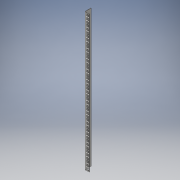
# Autodesk Inventor part: 15U_rack_strip
Saved by Autodesk Inventor 2016 (Build 200138000, 138)
## iProperties
Created: 2016-10-05
Part Number: 15U_rack_strip
Material: Generic
Document SubType Name: Sheet Metal
Designer: gmmar
Density: 1 g/cm^3
Sheet Metal Rule: Default
Appearance: Default
Author: gmmar
Autodesk Inventor part; units mm, degrees
ref_plane "YZ Plane" through (0, 0, 0) normal (1, 0, 0) x (0, 1, 0)
ref_plane "XZ Plane" through (0, 0, 0) normal (0, 1, 0) x (-1, 0, 0)
ref_plane "XY Plane" through (0, 0, 0) normal (0, 0, 1) x (1, 0, 0)
sketch "Sketch1" plane through (0, 0, 0) normal (0, 0, 1) x (1, 0, 0)
  line L0 (-22.7601, 80.4963) -> (27.2399, 80.4963)
  line L1 (27.2399, 80.4963) -> (27.2399, -590.5037)
  line L2 (27.2399, -590.5037) -> (-22.7601, -590.5037)
  line L3 (-22.7601, -590.5037) -> (-22.7601, 80.4963)
  line L4 (25.2399, 77.4963) -> (15.2399, 77.4963)
  line L5 (15.2399, 77.4963) -> (15.2399, 67.4963)
  line L6 (15.2399, 67.4963) -> (25.2399, 67.4963)
  line L7 (25.2399, 67.4963) -> (25.2399, 77.4963)
  line L8 (15.2399, 61.6213) -> (25.2399, 61.6213)
  line L9 (25.2399, 61.6213) -> (25.2399, 51.6213)
  line L10 (25.2399, 51.6213) -> (15.2399, 51.6213)
  line L11 (15.2399, 51.6213) -> (15.2399, 61.6213)
  line L12 (15.2399, 45.7463) -> (25.2399, 45.7463)
  line L13 (25.2399, 45.7463) -> (25.2399, 35.7463)
  line L14 (25.2399, 35.7463) -> (15.2399, 35.7463)
  line L15 (15.2399, 35.7463) -> (15.2399, 45.7463)
  line L16 (15.8399, 79.6042) -> (24.6399, 79.6042)
  line L17 (25.2399, 79.0042) -> (25.2399, 78.6883)
  line L18 (24.6399, 78.0883) -> (15.8399, 78.0883)
  line L19 (15.2399, 78.6883) -> (15.2399, 79.0042)
  line L20 (15.2399, 79.6042) -> (25.2399, 78.0883) construction
  line L21 (25.2399, 79.6042) -> (15.2399, 78.0883) construction
  arc A0 (15.8399, 79.6042) -> (15.2399, 79.0042) centre (15.8399, 79.0042) ccw
  arc A1 (15.2399, 78.6883) -> (15.8399, 78.0883) centre (15.8399, 78.6883) ccw
  arc A2 (24.6399, 78.0883) -> (25.2399, 78.6883) centre (24.6399, 78.6883) ccw
  arc A3 (25.2399, 79.0042) -> (24.6399, 79.6042) centre (24.6399, 79.0042) ccw
  circle A4 centre (-11.0789, 56.1463) radius 2.6
  line L22 (15.2399, 17.1713) -> (25.2399, 17.1713)
  circle A5 centre (-11.0789, 11.6963) radius 2.6
  line L23 (15.2399, 7.1713) -> (15.2399, 17.1713)
  line L24 (25.2399, 17.1713) -> (25.2399, 7.1713)
  line L25 (25.2399, 7.1713) -> (15.2399, 7.1713)
  line L26 (15.2399, 1.2963) -> (25.2399, 1.2963)
  line L27 (15.2399, -8.7037) -> (15.2399, 1.2963)
  line L28 (25.2399, -8.7037) -> (15.2399, -8.7037)
  line L29 (25.2399, 1.2963) -> (25.2399, -8.7037)
  line L30 (25.2399, 33.0463) -> (15.2399, 33.0463)
  line L31 (15.2399, 33.0463) -> (15.2399, 23.0463)
  line L32 (15.2399, 23.0463) -> (25.2399, 23.0463)
  line L33 (25.2399, 23.0463) -> (25.2399, 33.0463)
  line L34 (25.2399, 34.5542) -> (25.2399, 34.2383)
  arc A6 (25.2399, 34.5542) -> (24.6399, 35.1542) centre (24.6399, 34.5542) ccw
  arc A7 (24.6399, 33.6383) -> (25.2399, 34.2383) centre (24.6399, 34.2383) ccw
  line L35 (24.6399, 33.6383) -> (15.8399, 33.6383)
  arc A8 (15.2399, 34.2383) -> (15.8399, 33.6383) centre (15.8399, 34.2383) ccw
  line L36 (15.2399, 35.1542) -> (25.2399, 33.6383) construction
  line L37 (25.2399, 35.1542) -> (15.2399, 33.6383) construction
  line L38 (15.8399, 35.1542) -> (24.6399, 35.1542)
  line L39 (15.2399, 34.2383) -> (15.2399, 34.5542)
  arc A9 (15.8399, 35.1542) -> (15.2399, 34.5542) centre (15.8399, 34.5542) ccw
  line L40 (15.2399, -27.2787) -> (25.2399, -27.2787)
  circle A10 centre (-11.0789, -32.7537) radius 2.6
  line L41 (15.2399, -37.2787) -> (15.2399, -27.2787)
  line L42 (25.2399, -27.2787) -> (25.2399, -37.2787)
  line L43 (25.2399, -37.2787) -> (15.2399, -37.2787)
  line L44 (15.2399, -43.1537) -> (25.2399, -43.1537)
  line L45 (15.2399, -53.1537) -> (15.2399, -43.1537)
  line L46 (25.2399, -53.1537) -> (15.2399, -53.1537)
  line L47 (25.2399, -43.1537) -> (25.2399, -53.1537)
  line L48 (25.2399, -11.4037) -> (15.2399, -11.4037)
  line L49 (15.2399, -11.4037) -> (15.2399, -21.4037)
  line L50 (15.2399, -21.4037) -> (25.2399, -21.4037)
  line L51 (25.2399, -21.4037) -> (25.2399, -11.4037)
  line L52 (25.2399, -9.8958) -> (25.2399, -10.2117)
  arc A11 (25.2399, -9.8958) -> (24.6399, -9.2958) centre (24.6399, -9.8958) ccw
  arc A12 (24.6399, -10.8117) -> (25.2399, -10.2117) centre (24.6399, -10.2117) ccw
  line L53 (24.6399, -10.8117) -> (15.8399, -10.8117)
  arc A13 (15.2399, -10.2117) -> (15.8399, -10.8117) centre (15.8399, -10.2117) ccw
  line L54 (15.2399, -9.2958) -> (25.2399, -10.8117) construction
  line L55 (25.2399, -9.2958) -> (15.2399, -10.8117) construction
  line L56 (15.8399, -9.2958) -> (24.6399, -9.2958)
  line L57 (15.2399, -10.2117) -> (15.2399, -9.8958)
  arc A14 (15.8399, -9.2958) -> (15.2399, -9.8958) centre (15.8399, -9.8958) ccw
  line L58 (15.2399, -71.7287) -> (25.2399, -71.7287)
  circle A15 centre (-11.0789, -77.2037) radius 2.6
  line L59 (15.2399, -81.7287) -> (15.2399, -71.7287)
  line L60 (25.2399, -71.7287) -> (25.2399, -81.7287)
  line L61 (25.2399, -81.7287) -> (15.2399, -81.7287)
  line L62 (15.2399, -87.6037) -> (25.2399, -87.6037)
  line L63 (15.2399, -97.6037) -> (15.2399, -87.6037)
  line L64 (25.2399, -97.6037) -> (15.2399, -97.6037)
  line L65 (25.2399, -87.6037) -> (25.2399, -97.6037)
  line L66 (25.2399, -55.8537) -> (15.2399, -55.8537)
  line L67 (15.2399, -55.8537) -> (15.2399, -65.8537)
  line L68 (15.2399, -65.8537) -> (25.2399, -65.8537)
  line L69 (25.2399, -65.8537) -> (25.2399, -55.8537)
  line L70 (25.2399, -54.3458) -> (25.2399, -54.6617)
  arc A16 (25.2399, -54.3458) -> (24.6399, -53.7458) centre (24.6399, -54.3458) ccw
  arc A17 (24.6399, -55.2617) -> (25.2399, -54.6617) centre (24.6399, -54.6617) ccw
  line L71 (24.6399, -55.2617) -> (15.8399, -55.2617)
  arc A18 (15.2399, -54.6617) -> (15.8399, -55.2617) centre (15.8399, -54.6617) ccw
  line L72 (15.2399, -53.7458) -> (25.2399, -55.2617) construction
  line L73 (25.2399, -53.7458) -> (15.2399, -55.2617) construction
  line L74 (15.8399, -53.7458) -> (24.6399, -53.7458)
  line L75 (15.2399, -54.6617) -> (15.2399, -54.3458)
  arc A19 (15.8399, -53.7458) -> (15.2399, -54.3458) centre (15.8399, -54.3458) ccw
  line L76 (15.2399, -116.1787) -> (25.2399, -116.1787)
  circle A20 centre (-11.0789, -121.6537) radius 2.6
  line L77 (15.2399, -126.1787) -> (15.2399, -116.1787)
  line L78 (25.2399, -116.1787) -> (25.2399, -126.1787)
  line L79 (25.2399, -126.1787) -> (15.2399, -126.1787)
  line L80 (15.2399, -132.0537) -> (25.2399, -132.0537)
  line L81 (15.2399, -142.0537) -> (15.2399, -132.0537)
  line L82 (25.2399, -142.0537) -> (15.2399, -142.0537)
  line L83 (25.2399, -132.0537) -> (25.2399, -142.0537)
  line L84 (25.2399, -100.3037) -> (15.2399, -100.3037)
  line L85 (15.2399, -100.3037) -> (15.2399, -110.3037)
  line L86 (15.2399, -110.3037) -> (25.2399, -110.3037)
  line L87 (25.2399, -110.3037) -> (25.2399, -100.3037)
  line L88 (25.2399, -98.7958) -> (25.2399, -99.1117)
  arc A21 (25.2399, -98.7958) -> (24.6399, -98.1958) centre (24.6399, -98.7958) ccw
  arc A22 (24.6399, -99.7117) -> (25.2399, -99.1117) centre (24.6399, -99.1117) ccw
  line L89 (24.6399, -99.7117) -> (15.8399, -99.7117)
  arc A23 (15.2399, -99.1117) -> (15.8399, -99.7117) centre (15.8399, -99.1117) ccw
  line L90 (15.2399, -98.1958) -> (25.2399, -99.7117) construction
  line L91 (25.2399, -98.1958) -> (15.2399, -99.7117) construction
  line L92 (15.8399, -98.1958) -> (24.6399, -98.1958)
  line L93 (15.2399, -99.1117) -> (15.2399, -98.7958)
  arc A24 (15.8399, -98.1958) -> (15.2399, -98.7958) centre (15.8399, -98.7958) ccw
  line L94 (15.2399, -160.6287) -> (25.2399, -160.6287)
  circle A25 centre (-11.0789, -166.1037) radius 2.6
  line L95 (15.2399, -170.6287) -> (15.2399, -160.6287)
  line L96 (25.2399, -160.6287) -> (25.2399, -170.6287)
  line L97 (25.2399, -170.6287) -> (15.2399, -170.6287)
  line L98 (15.2399, -176.5037) -> (25.2399, -176.5037)
  line L99 (15.2399, -186.5037) -> (15.2399, -176.5037)
  line L100 (25.2399, -186.5037) -> (15.2399, -186.5037)
  line L101 (25.2399, -176.5037) -> (25.2399, -186.5037)
  line L102 (25.2399, -144.7537) -> (15.2399, -144.7537)
  line L103 (15.2399, -144.7537) -> (15.2399, -154.7537)
  line L104 (15.2399, -154.7537) -> (25.2399, -154.7537)
  line L105 (25.2399, -154.7537) -> (25.2399, -144.7537)
  line L106 (25.2399, -143.2458) -> (25.2399, -143.5617)
  arc A26 (25.2399, -143.2458) -> (24.6399, -142.6458) centre (24.6399, -143.2458) ccw
  arc A27 (24.6399, -144.1617) -> (25.2399, -143.5617) centre (24.6399, -143.5617) ccw
  line L107 (24.6399, -144.1617) -> (15.8399, -144.1617)
  arc A28 (15.2399, -143.5617) -> (15.8399, -144.1617) centre (15.8399, -143.5617) ccw
  line L108 (15.2399, -142.6458) -> (25.2399, -144.1617) construction
  line L109 (25.2399, -142.6458) -> (15.2399, -144.1617) construction
  line L110 (15.8399, -142.6458) -> (24.6399, -142.6458)
  line L111 (15.2399, -143.5617) -> (15.2399, -143.2458)
  arc A29 (15.8399, -142.6458) -> (15.2399, -143.2458) centre (15.8399, -143.2458) ccw
  line L112 (15.2399, -205.0787) -> (25.2399, -205.0787)
  circle A30 centre (-11.0789, -210.5537) radius 2.6
  line L113 (15.2399, -215.0787) -> (15.2399, -205.0787)
  line L114 (25.2399, -205.0787) -> (25.2399, -215.0787)
  line L115 (25.2399, -215.0787) -> (15.2399, -215.0787)
  line L116 (15.2399, -220.9537) -> (25.2399, -220.9537)
  line L117 (15.2399, -230.9537) -> (15.2399, -220.9537)
  line L118 (25.2399, -230.9537) -> (15.2399, -230.9537)
  line L119 (25.2399, -220.9537) -> (25.2399, -230.9537)
  line L120 (25.2399, -189.2037) -> (15.2399, -189.2037)
  line L121 (15.2399, -189.2037) -> (15.2399, -199.2037)
  line L122 (15.2399, -199.2037) -> (25.2399, -199.2037)
  line L123 (25.2399, -199.2037) -> (25.2399, -189.2037)
  line L124 (25.2399, -187.6958) -> (25.2399, -188.0117)
  arc A31 (25.2399, -187.6958) -> (24.6399, -187.0958) centre (24.6399, -187.6958) ccw
  arc A32 (24.6399, -188.6117) -> (25.2399, -188.0117) centre (24.6399, -188.0117) ccw
  line L125 (24.6399, -188.6117) -> (15.8399, -188.6117)
  arc A33 (15.2399, -188.0117) -> (15.8399, -188.6117) centre (15.8399, -188.0117) ccw
  line L126 (15.2399, -187.0958) -> (25.2399, -188.6117) construction
  line L127 (25.2399, -187.0958) -> (15.2399, -188.6117) construction
  line L128 (15.8399, -187.0958) -> (24.6399, -187.0958)
  line L129 (15.2399, -188.0117) -> (15.2399, -187.6958)
  arc A34 (15.8399, -187.0958) -> (15.2399, -187.6958) centre (15.8399, -187.6958) ccw
  line L130 (15.2399, -249.5287) -> (25.2399, -249.5287)
  circle A35 centre (-11.0789, -255.0037) radius 2.6
  line L131 (15.2399, -259.5287) -> (15.2399, -249.5287)
  line L132 (25.2399, -249.5287) -> (25.2399, -259.5287)
  line L133 (25.2399, -259.5287) -> (15.2399, -259.5287)
  line L134 (15.2399, -265.4037) -> (25.2399, -265.4037)
  line L135 (15.2399, -275.4037) -> (15.2399, -265.4037)
  line L136 (25.2399, -275.4037) -> (15.2399, -275.4037)
  line L137 (25.2399, -265.4037) -> (25.2399, -275.4037)
  line L138 (25.2399, -233.6537) -> (15.2399, -233.6537)
  line L139 (15.2399, -233.6537) -> (15.2399, -243.6537)
  line L140 (15.2399, -243.6537) -> (25.2399, -243.6537)
  line L141 (25.2399, -243.6537) -> (25.2399, -233.6537)
  line L142 (25.2399, -232.1458) -> (25.2399, -232.4617)
  arc A36 (25.2399, -232.1458) -> (24.6399, -231.5458) centre (24.6399, -232.1458) ccw
  arc A37 (24.6399, -233.0617) -> (25.2399, -232.4617) centre (24.6399, -232.4617) ccw
  line L143 (24.6399, -233.0617) -> (15.8399, -233.0617)
  arc A38 (15.2399, -232.4617) -> (15.8399, -233.0617) centre (15.8399, -232.4617) ccw
  line L144 (15.2399, -231.5458) -> (25.2399, -233.0617) construction
  line L145 (25.2399, -231.5458) -> (15.2399, -233.0617) construction
  line L146 (15.8399, -231.5458) -> (24.6399, -231.5458)
  line L147 (15.2399, -232.4617) -> (15.2399, -232.1458)
  arc A39 (15.8399, -231.5458) -> (15.2399, -232.1458) centre (15.8399, -232.1458) ccw
  line L148 (15.2399, -293.9787) -> (25.2399, -293.9787)
  circle A40 centre (-11.0789, -299.4537) radius 2.6
  line L149 (15.2399, -303.9787) -> (15.2399, -293.9787)
  line L150 (25.2399, -293.9787) -> (25.2399, -303.9787)
  line L151 (25.2399, -303.9787) -> (15.2399, -303.9787)
  line L152 (15.2399, -309.8537) -> (25.2399, -309.8537)
  line L153 (15.2399, -319.8537) -> (15.2399, -309.8537)
  line L154 (25.2399, -319.8537) -> (15.2399, -319.8537)
  line L155 (25.2399, -309.8537) -> (25.2399, -319.8537)
  line L156 (25.2399, -278.1037) -> (15.2399, -278.1037)
  line L157 (15.2399, -278.1037) -> (15.2399, -288.1037)
  line L158 (15.2399, -288.1037) -> (25.2399, -288.1037)
  line L159 (25.2399, -288.1037) -> (25.2399, -278.1037)
  line L160 (25.2399, -276.5958) -> (25.2399, -276.9117)
  arc A41 (25.2399, -276.5958) -> (24.6399, -275.9958) centre (24.6399, -276.5958) ccw
  arc A42 (24.6399, -277.5117) -> (25.2399, -276.9117) centre (24.6399, -276.9117) ccw
  line L161 (24.6399, -277.5117) -> (15.8399, -277.5117)
  arc A43 (15.2399, -276.9117) -> (15.8399, -277.5117) centre (15.8399, -276.9117) ccw
  line L162 (15.2399, -275.9958) -> (25.2399, -277.5117) construction
  line L163 (25.2399, -275.9958) -> (15.2399, -277.5117) construction
  line L164 (15.8399, -275.9958) -> (24.6399, -275.9958)
  line L165 (15.2399, -276.9117) -> (15.2399, -276.5958)
  arc A44 (15.8399, -275.9958) -> (15.2399, -276.5958) centre (15.8399, -276.5958) ccw
  line L166 (15.2399, -338.4287) -> (25.2399, -338.4287)
  circle A45 centre (-11.0789, -343.9037) radius 2.6
  line L167 (15.2399, -348.4287) -> (15.2399, -338.4287)
  line L168 (25.2399, -338.4287) -> (25.2399, -348.4287)
  line L169 (25.2399, -348.4287) -> (15.2399, -348.4287)
  line L170 (15.2399, -354.3037) -> (25.2399, -354.3037)
  line L171 (15.2399, -364.3037) -> (15.2399, -354.3037)
  line L172 (25.2399, -364.3037) -> (15.2399, -364.3037)
  line L173 (25.2399, -354.3037) -> (25.2399, -364.3037)
  line L174 (25.2399, -322.5537) -> (15.2399, -322.5537)
  line L175 (15.2399, -322.5537) -> (15.2399, -332.5537)
  line L176 (15.2399, -332.5537) -> (25.2399, -332.5537)
  line L177 (25.2399, -332.5537) -> (25.2399, -322.5537)
  line L178 (25.2399, -321.0458) -> (25.2399, -321.3617)
  arc A46 (25.2399, -321.0458) -> (24.6399, -320.4458) centre (24.6399, -321.0458) ccw
  arc A47 (24.6399, -321.9617) -> (25.2399, -321.3617) centre (24.6399, -321.3617) ccw
  line L179 (24.6399, -321.9617) -> (15.8399, -321.9617)
  arc A48 (15.2399, -321.3617) -> (15.8399, -321.9617) centre (15.8399, -321.3617) ccw
  line L180 (15.2399, -320.4458) -> (25.2399, -321.9617) construction
  line L181 (25.2399, -320.4458) -> (15.2399, -321.9617) construction
  line L182 (15.8399, -320.4458) -> (24.6399, -320.4458)
  line L183 (15.2399, -321.3617) -> (15.2399, -321.0458)
  arc A49 (15.8399, -320.4458) -> (15.2399, -321.0458) centre (15.8399, -321.0458) ccw
  line L184 (15.2399, -382.8787) -> (25.2399, -382.8787)
  circle A50 centre (-11.0789, -388.3537) radius 2.6
  line L185 (15.2399, -392.8787) -> (15.2399, -382.8787)
  line L186 (25.2399, -382.8787) -> (25.2399, -392.8787)
  line L187 (25.2399, -392.8787) -> (15.2399, -392.8787)
  line L188 (15.2399, -398.7537) -> (25.2399, -398.7537)
  line L189 (15.2399, -408.7537) -> (15.2399, -398.7537)
  line L190 (25.2399, -408.7537) -> (15.2399, -408.7537)
  line L191 (25.2399, -398.7537) -> (25.2399, -408.7537)
  line L192 (25.2399, -367.0037) -> (15.2399, -367.0037)
  line L193 (15.2399, -367.0037) -> (15.2399, -377.0037)
  line L194 (15.2399, -377.0037) -> (25.2399, -377.0037)
  line L195 (25.2399, -377.0037) -> (25.2399, -367.0037)
  line L196 (25.2399, -365.4958) -> (25.2399, -365.8117)
  arc A51 (25.2399, -365.4958) -> (24.6399, -364.8958) centre (24.6399, -365.4958) ccw
  arc A52 (24.6399, -366.4117) -> (25.2399, -365.8117) centre (24.6399, -365.8117) ccw
  line L197 (24.6399, -366.4117) -> (15.8399, -366.4117)
  arc A53 (15.2399, -365.8117) -> (15.8399, -366.4117) centre (15.8399, -365.8117) ccw
  line L198 (15.2399, -364.8958) -> (25.2399, -366.4117) construction
  line L199 (25.2399, -364.8958) -> (15.2399, -366.4117) construction
  line L200 (15.8399, -364.8958) -> (24.6399, -364.8958)
  line L201 (15.2399, -365.8117) -> (15.2399, -365.4958)
  arc A54 (15.8399, -364.8958) -> (15.2399, -365.4958) centre (15.8399, -365.4958) ccw
  line L202 (15.2399, -427.3287) -> (25.2399, -427.3287)
  circle A55 centre (-11.0789, -432.8037) radius 2.6
  line L203 (15.2399, -437.3287) -> (15.2399, -427.3287)
  line L204 (25.2399, -427.3287) -> (25.2399, -437.3287)
  line L205 (25.2399, -437.3287) -> (15.2399, -437.3287)
  line L206 (15.2399, -443.2037) -> (25.2399, -443.2037)
  line L207 (15.2399, -453.2037) -> (15.2399, -443.2037)
  line L208 (25.2399, -453.2037) -> (15.2399, -453.2037)
  line L209 (25.2399, -443.2037) -> (25.2399, -453.2037)
  line L210 (25.2399, -411.4537) -> (15.2399, -411.4537)
  line L211 (15.2399, -411.4537) -> (15.2399, -421.4537)
  line L212 (15.2399, -421.4537) -> (25.2399, -421.4537)
  line L213 (25.2399, -421.4537) -> (25.2399, -411.4537)
  line L214 (25.2399, -409.9458) -> (25.2399, -410.2617)
  arc A56 (25.2399, -409.9458) -> (24.6399, -409.3458) centre (24.6399, -409.9458) ccw
  arc A57 (24.6399, -410.8617) -> (25.2399, -410.2617) centre (24.6399, -410.2617) ccw
  line L215 (24.6399, -410.8617) -> (15.8399, -410.8617)
  arc A58 (15.2399, -410.2617) -> (15.8399, -410.8617) centre (15.8399, -410.2617) ccw
  line L216 (15.2399, -409.3458) -> (25.2399, -410.8617) construction
  line L217 (25.2399, -409.3458) -> (15.2399, -410.8617) construction
  line L218 (15.8399, -409.3458) -> (24.6399, -409.3458)
  line L219 (15.2399, -410.2617) -> (15.2399, -409.9458)
  arc A59 (15.8399, -409.3458) -> (15.2399, -409.9458) centre (15.8399, -409.9458) ccw
  line L220 (15.2399, -471.7787) -> (25.2399, -471.7787)
  circle A60 centre (-11.0789, -477.2537) radius 2.6
  line L221 (15.2399, -481.7787) -> (15.2399, -471.7787)
  line L222 (25.2399, -471.7787) -> (25.2399, -481.7787)
  line L223 (25.2399, -481.7787) -> (15.2399, -481.7787)
  line L224 (15.2399, -487.6537) -> (25.2399, -487.6537)
  line L225 (15.2399, -497.6537) -> (15.2399, -487.6537)
  line L226 (25.2399, -497.6537) -> (15.2399, -497.6537)
  line L227 (25.2399, -487.6537) -> (25.2399, -497.6537)
  line L228 (25.2399, -455.9037) -> (15.2399, -455.9037)
  line L229 (15.2399, -455.9037) -> (15.2399, -465.9037)
  line L230 (15.2399, -465.9037) -> (25.2399, -465.9037)
  line L231 (25.2399, -465.9037) -> (25.2399, -455.9037)
  line L232 (25.2399, -454.3958) -> (25.2399, -454.7117)
  arc A61 (25.2399, -454.3958) -> (24.6399, -453.7958) centre (24.6399, -454.3958) ccw
  arc A62 (24.6399, -455.3117) -> (25.2399, -454.7117) centre (24.6399, -454.7117) ccw
  line L233 (24.6399, -455.3117) -> (15.8399, -455.3117)
  arc A63 (15.2399, -454.7117) -> (15.8399, -455.3117) centre (15.8399, -454.7117) ccw
  line L234 (15.2399, -453.7958) -> (25.2399, -455.3117) construction
  line L235 (25.2399, -453.7958) -> (15.2399, -455.3117) construction
  line L236 (15.8399, -453.7958) -> (24.6399, -453.7958)
  line L237 (15.2399, -454.7117) -> (15.2399, -454.3958)
  arc A64 (15.8399, -453.7958) -> (15.2399, -454.3958) centre (15.8399, -454.3958) ccw
  line L238 (15.2399, -516.2287) -> (25.2399, -516.2287)
  circle A65 centre (-11.0789, -521.7037) radius 2.6
  line L239 (15.2399, -526.2287) -> (15.2399, -516.2287)
  line L240 (25.2399, -516.2287) -> (25.2399, -526.2287)
  line L241 (25.2399, -526.2287) -> (15.2399, -526.2287)
  line L242 (15.2399, -532.1037) -> (25.2399, -532.1037)
  line L243 (15.2399, -542.1037) -> (15.2399, -532.1037)
  line L244 (25.2399, -542.1037) -> (15.2399, -542.1037)
  line L245 (25.2399, -532.1037) -> (25.2399, -542.1037)
  line L246 (25.2399, -500.3537) -> (15.2399, -500.3537)
  line L247 (15.2399, -500.3537) -> (15.2399, -510.3537)
  line L248 (15.2399, -510.3537) -> (25.2399, -510.3537)
  line L249 (25.2399, -510.3537) -> (25.2399, -500.3537)
  line L250 (25.2399, -498.8458) -> (25.2399, -499.1617)
  arc A66 (25.2399, -498.8458) -> (24.6399, -498.2458) centre (24.6399, -498.8458) ccw
  arc A67 (24.6399, -499.7617) -> (25.2399, -499.1617) centre (24.6399, -499.1617) ccw
  line L251 (24.6399, -499.7617) -> (15.8399, -499.7617)
  arc A68 (15.2399, -499.1617) -> (15.8399, -499.7617) centre (15.8399, -499.1617) ccw
  line L252 (15.2399, -498.2458) -> (25.2399, -499.7617) construction
  line L253 (25.2399, -498.2458) -> (15.2399, -499.7617) construction
  line L254 (15.8399, -498.2458) -> (24.6399, -498.2458)
  line L255 (15.2399, -499.1617) -> (15.2399, -498.8458)
  arc A69 (15.8399, -498.2458) -> (15.2399, -498.8458) centre (15.8399, -498.8458) ccw
  line L256 (15.2399, -560.6787) -> (25.2399, -560.6787)
  circle A70 centre (-11.0789, -566.1537) radius 2.6
  line L257 (15.2399, -570.6787) -> (15.2399, -560.6787)
  line L258 (25.2399, -560.6787) -> (25.2399, -570.6787)
  line L259 (25.2399, -570.6787) -> (15.2399, -570.6787)
  line L260 (15.2399, -576.5537) -> (25.2399, -576.5537)
  line L261 (15.2399, -586.5537) -> (15.2399, -576.5537)
  line L262 (25.2399, -586.5537) -> (15.2399, -586.5537)
  line L263 (25.2399, -576.5537) -> (25.2399, -586.5537)
  line L264 (25.2399, -544.8037) -> (15.2399, -544.8037)
  line L265 (15.2399, -544.8037) -> (15.2399, -554.8037)
  line L266 (15.2399, -554.8037) -> (25.2399, -554.8037)
  line L267 (25.2399, -554.8037) -> (25.2399, -544.8037)
  line L268 (25.2399, -543.2958) -> (25.2399, -543.6117)
  arc A71 (25.2399, -543.2958) -> (24.6399, -542.6958) centre (24.6399, -543.2958) ccw
  arc A72 (24.6399, -544.2117) -> (25.2399, -543.6117) centre (24.6399, -543.6117) ccw
  line L269 (24.6399, -544.2117) -> (15.8399, -544.2117)
  arc A73 (15.2399, -543.6117) -> (15.8399, -544.2117) centre (15.8399, -543.6117) ccw
  line L270 (15.2399, -542.6958) -> (25.2399, -544.2117) construction
  line L271 (25.2399, -542.6958) -> (15.2399, -544.2117) construction
  line L272 (15.8399, -542.6958) -> (24.6399, -542.6958)
  line L273 (15.2399, -543.6117) -> (15.2399, -543.2958)
  arc A74 (15.8399, -542.6958) -> (15.2399, -543.2958) centre (15.8399, -543.2958) ccw
  point P0 (0, 0)
  point P1 (20.2399, 78.8463)
  point P2 (20.2399, 34.3963)
  point P3 (20.2399, -10.0537)
  point P4 (20.2399, -54.5037)
  point P5 (20.2399, -98.9537)
  point P6 (20.2399, -143.4037)
  point P7 (20.2399, -187.8537)
  point P8 (20.2399, -232.3037)
  point P9 (20.2399, -276.7537)
  point P10 (20.2399, -321.2037)
  point P11 (20.2399, -365.6537)
  point P12 (20.2399, -410.1037)
  point P13 (20.2399, -454.5537)
  point P14 (20.2399, -499.0037)
  point P15 (20.2399, -543.4537)
  dimension "d0" = 50
  dimension "d1" = 671
  dimension "d2" = 10
  dimension "d3" = 10
  dimension "d4" = 10
  dimension "d5" = 10
  dimension "d8" = 3
  dimension "d9" = 2
  dimension "d10" = 1.35
  dimension "d11" = 0.6
  dimension "d12" = 0.6
  dimension "d13" = 0.6
  dimension "d14" = 0.6
  dimension "d21" = 2
  dimension "d22" = 10
  dimension "d23" = 5.2
  dimension "d24" = 11.6813
  dimension "d25" = 41.75
  dimension "d26" = 5.875
  dimension "d27" = 5.875
  dimension "d30" = 44.45
  measures "d0" distance of L0.start L0.end
  measures "d1" distance of L0.end L1.end
  measures "d2" distance of L6.end L5.end
  measures "d3" distance of L5.end L4.end
  measures "d4" distance of L8.end L9.end
  measures "d5" distance of L12.end L13.end
  measures "d8" distance between parallel lines of L0 L4
  measures "d9" distance between parallel lines of L1 L7
  measures "d10" distance from line of L4 point (20.24, 78.846)
  measures "d11" radius of A0
  measures "d12" radius of A1
  measures "d13" radius of A2
  measures "d14" radius of A3
  measures "d21" distance between parallel lines of L1 L13
  measures "d22" distance between parallel lines of L13 L15
  measures "d23" diameter of A4
  measures "d24" distance from line of L3 A4.centre
  measures "d25" distance between parallel lines of L14 L4
  measures "d26" distance between parallel lines of L8 L6
  measures "d27" distance between parallel lines of L12 L10
  measures "d30" distance of A4.centre A5.centre
extrude "Plate1" add sketch "Sketch1" against normal blind 2 contours L0 L1 L2 L3 | L16 A3 L17 A2 L18 A1 L19 A0 | L34 A7 L35 A8 L39 A9 L38 A6 | L52 A12 L53 A13 L57 A14 L56 A11 | L70 A17 L71 A18 L75 A19 L74 A16 | L88 A22 L89 A23 L93 A24 L92 A21 | L106 A27 L107 A28 L111 A29 L110 A26 | L124 A32 L125 A33 L129 A34 L128 A31 | L142 A37 L143 A38 L147 A39 L146 A36 | L160 A42 L161 A43 L165 A44 L164 A41 | L178 A47 L179 A48 L183 A49 L182 A46 | L196 A52 L197 A53 L201 A54 L200 A51 | L214 A57 L215 A58 L219 A59 L218 A56 | L232 A62 L233 A63 L237 A64 L236 A61 | L250 A67 L251 A68 L255 A69 L254 A66 | L268 A72 L269 A73 L273 A74 L272 A71
sketch "Sketch4" plane through (0, 0, 0) normal (0, 0, 1) x (1, 0, 0)
  line L0 (-22.7601, 80.4963) -> (27.2399, 80.4963) projected
  line L1 (6.7399, 80.4963) -> (6.7399, -590.5037)
  line L2 (27.2399, -590.5037) -> (-22.7601, -590.5037) projected
  line L3 (-22.7601, 80.4963) -> (-22.7601, -590.5037) projected
  point P0 (0, 0)
  dimension "d37" = 29.5
  constraints: 2 end point, 2 point on line, 1 vertical
  measures "d37" distance between parallel lines of L3 L1
fold "Fold1" angle 90 bend radius 2.5 thickness 2 k factor 0.44 line from (6.7399, 80.4963, 0) to (6.7399, -590.5037, 0) line at bend centre moving side (-1, 0, 0) folds toward (0, 0, -1)
equation "\"d38\" = BendReliefWidth"
equation "\"d39\" = BendReliefDepth"
equation "\"d40\" = MinimumRemnant"
equation "\"d41\" = BendRadius"
equation "\"BendRadius\" = Thickness"
equation "\"BendReliefWidth\" = Thickness"
equation "\"BendReliefDepth\" = 0.5 * Thickness"
equation "\"CornerReliefSize\" = 4 * Thickness"
equation "\"MinimumRemnant\" = 2 * Thickness"
equation "\"TransitionRadius\" = BendRadius"
equation "\"JacobiRadiusSize\" = BendRadius"
equation "\"GapSize\" = Thickness"
equation "\"d35\" = BendRadius"
equation "\"Thickness\" = 2"
body "Solid1"
